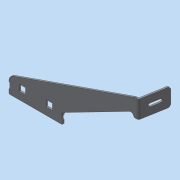
# Autodesk Inventor part: 0 零件
Saved by Autodesk Inventor 2020 (Build 240168000, 168)
## iProperties
Created: 2020-11-03
Part Number: 0 零件
Material: 一般
Document SubType Name: Modeling
Designer: p2013
Density: 1 g/cm^3
Appearance: 預設
Author: p2013
Autodesk Inventor part; units mm, degrees
ref_plane "YZ Plane" through (0, 0, 0) normal (1, 0, 0) x (0, 1, 0)
ref_plane "XZ Plane" through (0, 0, 0) normal (0, 1, 0) x (-1, 0, 0)
ref_plane "XY Plane" through (0, 0, 0) normal (0, 0, 1) x (1, 0, 0)
sketch "草圖1" plane through (0, 0, 0) normal (0, 0, 1) x (1, 0, 0)
  line L0 (0, 0) -> (-7.8042, 0) construction
  line L1 (0, 0) -> (0, -16.694) construction
  line L2 (0, 2) -> (0, 28)
  line L3 (310, 145) -> (310, 102)
  line L4 (130, 19.7875) -> (130, 2)
  line L5 (128, 0) -> (2, 0)
  line L6 (310, 145) -> (368, 145)
  line L7 (375, 138) -> (375, 109)
  line L8 (368, 102) -> (310, 102)
  line L9 (332, 127.5) -> (354, 127.5)
  arc A0 (354, 119.5) -> (354, 127.5) centre (354, 123.5) ccw
  line L10 (354, 119.5) -> (332, 119.5)
  arc A1 (332, 127.5) -> (332, 119.5) centre (332, 123.5) ccw
  line L11 (65, 14) -> (65, 14) construction
  arc A2 (10.0615, 42.1637) -> (0, 28) centre (15, 28) ccw
  line L12 (10.0615, 42.1637) -> (303.401, 144.4425)
  line L13 (306.6934, 145) -> (310, 145)
  line L14 (310, 102) -> (305, 102)
  line L15 (291.9999, 109.2247) -> (135.4256, 28.6799)
  arc A3 (375, 138) -> (368, 145) centre (368, 138) ccw
  arc A4 (368, 102) -> (375, 109) centre (368, 109) ccw
  arc A5 (302.0606, 104.4) -> (305, 102) centre (305, 105) ccw
  arc A6 (302.0606, 104.4) -> (291.9999, 109.2247) centre (295.202, 103) ccw
  arc A7 (306.6934, 145) -> (303.401, 144.4425) centre (306.6934, 135) ccw
  arc A8 (135.4256, 28.6799) -> (130, 19.7875) centre (140, 19.7875) ccw
  line L16 (24.9, 33) -> (40.1, 33)
  line L17 (40.1, 33) -> (40.1, 18)
  line L18 (40.1, 18) -> (24.9, 18)
  line L19 (24.9, 18) -> (24.9, 33)
  line L20 (89.9, 33) -> (105.1, 33)
  line L21 (105.1, 33) -> (105.1, 18)
  line L22 (105.1, 18) -> (89.9, 18)
  line L23 (89.9, 18) -> (89.9, 33)
  line L24 (40.1, 25.5) -> (89.9, 25.5) construction
  line L25 (0, 25.2) -> (2, 25.2)
  line L26 (2, 25.2) -> (2, 10.2)
  line L27 (2, 10.2) -> (0, 10.2)
  line L28 (0, 10.2) -> (0, 25.2)
  line L29 (65, 0) -> (65, 25.5) construction
  line L30 (130, 25.2) -> (128, 25.2)
  line L31 (128, 25.2) -> (128, 10.2)
  line L32 (128, 10.2) -> (130, 10.2)
  line L33 (130, 10.2) -> (130, 25.2)
  arc A9 (0, 2) -> (2, 0) centre (2, 2) ccw
  arc A10 (128, 0) -> (130, 2) centre (128, 2) ccw
  point P0 (130, 0)
  point P1 (375, 145)
  point P2 (375, 102)
  point P3 (130, 25.8889)
  point P4 (305, 145)
  point P5 (305, 102)
  point P6 (305, 115.9121)
  point P7 (32.5, 33)
  point P8 (97.5, 33)
  point P9 (0, 10.2)
  point P10 (130, 28)
  dimension "d0" = 130
  dimension "d1" = 145
  dimension "d2" = 43
  dimension "d3" = 65
  dimension "d4" = 8
  dimension "d5" = 30
  dimension "d7" = 18
  dimension "d8" = 310
  dimension "d14" = 14
  dimension "d17" = 21.5
  dimension "d20" = 15
  dimension "d21" = 28
  dimension "d23" = 5
  dimension "d24" = 7
  dimension "d26" = 3
  dimension "d28" = 35
  dimension "d29" = 7
  dimension "d30" = 5
  dimension "d31" = 10
  dimension "d32" = 10
  dimension "d33" = 8
  dimension "d34" = 15.2
  dimension "d35" = 15.2
  dimension "d36" = 15
  dimension "d37" = 65
  dimension "d38" = 33
  dimension "d39" = 15
  dimension "d40" = 2
  dimension "d41" = 10.2
  dimension "d42" = 2
  constraints: 69 end point, 23 point on circle, 21 tangent, 15 point on line, 11 centre point, 9 horizontal, 9 parallel, 7 midpoint, 6 perpendicular, 5 symmetric about line, 5 vertical alignment, 3 vertical, 2 collinear, 2 equal radius, 1 coincident
  measures "d0" distance between parallel lines of L4 L2
  measures "d1" distance from line of L3.start L5
  measures "d2" distance between parallel lines of L6 L8
  measures "d3" distance between parallel lines of L7 L3
  measures "d4" distance between parallel lines of L10 L9
  measures "d7" distance edge to line of A1 L3
  measures "d8" distance between parallel lines of L3 L2
  measures "d14" distance from line of L5 L11.start
  measures "d17" distance from line of L6 A0.centre
  measures "d20" radius of A2
  measures "d21" distance of L0.start L2.end
  measures "d23" distance of point (305, 145) L3.start
  measures "d24" radius of A3
  measures "d26" radius of A5
  measures "d28" distance edge to line of A6 L13
  measures "d29" radius of A6
  measures "d30" distance of L3.end L14.end
  measures "d31" radius of A7
  measures "d32" radius of A8
  measures "d33" angle of L15 L12
  measures "d34" distance between parallel lines of L17 L19
  measures "d35" distance between parallel lines of L21 L23
  measures "d36" distance between parallel lines of L16 L18
  measures "d37" distance of point (32.5, 33) point (97.5, 33)
  measures "d38" distance between parallel lines of L5 L16
  measures "d39" distance between parallel lines of L27 L25
  measures "d40" distance between parallel lines of L28 L26
  measures "d41" distance between parallel lines of L27 L5
  measures "d42" radius of A9
extrude "擠出1" add sketch "草圖1" along normal blind 3.5 contours L2 L27 L26 L25 A2 L12 A7 L13 L3 L14 A5 A6 L15 A8 L33 L30 L31 L32 L4 A10 L5 A9 | L6 A3 L7 A4 L8 L3
bend part "折彎零件1" radius 0.5 angle 80 line through (310, 145, 0) along (0, -1, 0) centre toward (0, 0, -1) moving side (1, 0, 0) both sides no
ref_plane "工作平面1" through (65, 0, 0) normal (-1, 0, 0) x (0, 0, 1)
